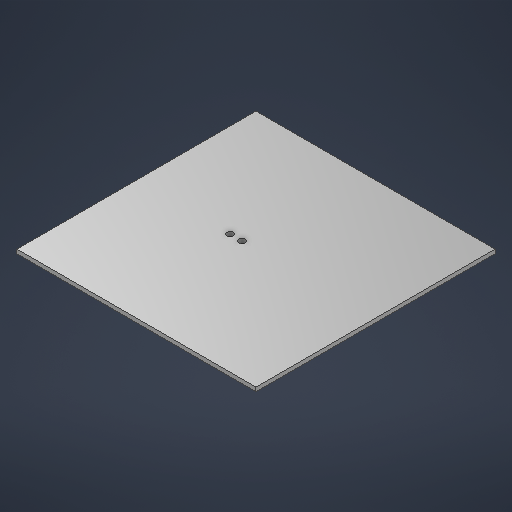
# Autodesk Inventor part: PlataformaLoadCell
Saved by Autodesk Inventor 2027 (Build 310192060, 192F)
## iProperties
Created: 2026-09-27
Part Number: PlataformaLoadCell
Material: PC/ABS Plastic
Document SubType Name: Modeling
Designer: notra
Density: 1.1 g/cm^3
Appearance: Smooth - White
Mass: 229.26 g
Surface Area: 860.831 cm^2
Volume: 208.419 cm^3
Author: notra
Autodesk Inventor part; units mm, degrees
ref_plane "YZ Plane" through (0, 0, 0) normal (1, 0, 0) x (0, 1, 0)
ref_plane "XZ Plane" through (0, 0, 0) normal (0, 1, 0) x (-1, 0, 0)
ref_plane "XY Plane" through (0, 0, 0) normal (0, 0, 1) x (1, 0, 0)
sketch "Sketch1" plane through (0, 0, 0) normal (0, 1, 0) x (-1, 0, 0)
  line L0 (-150, 150) -> (150, 150)
  line L1 (150, 150) -> (150, -150)
  line L2 (150, -150) -> (-150, -150)
  line L3 (-150, -150) -> (-150, 150)
  line L4 (-150, 150) -> (150, -150) construction
  line L5 (150, 150) -> (-150, -150) construction
  line L6 (150, 0) -> (-150, 0) construction
  line L7 (0, 150) -> (0, -150) construction
  line L8 (37.5, 6.35) -> (-37.5, 6.35) construction
  line L9 (-37.5, 6.35) -> (-37.5, -6.35) construction
  line L10 (-37.5, -6.35) -> (37.5, -6.35) construction
  line L11 (37.5, -6.35) -> (37.5, 6.35) construction
  line L12 (37.5, 6.35) -> (-37.5, -6.35) construction
  line L13 (-37.5, 6.35) -> (37.5, -6.35) construction
  circle A0 centre (32.5, 0) radius 2
  circle A1 centre (17.5, 0) radius 2
  circle A2 centre (-32.5, 0) radius 2 construction
  circle A3 centre (-17.5, 0) radius 2 construction
  line L14 (30.5, 0) -> (19.5, 0) construction
  line L15 (42.5, 13.75) -> (7.5, 13.75)
  line L16 (7.5, 13.75) -> (7.5, -13.75)
  line L17 (7.5, -13.75) -> (42.5, -13.75)
  line L18 (42.5, -13.75) -> (42.5, 13.75)
  line L19 (42.5, 13.75) -> (7.5, -13.75) construction
  line L20 (7.5, 13.75) -> (42.5, -13.75) construction
  circle A4 centre (32.5, 0) radius 4
  circle A5 centre (17.5, 0) radius 4
  point P0 (0, 0)
  point P1 (37.5, 0)
  point P2 (25, 0)
  dimension "d4" = 4
  dimension "d7" = 4
  dimension "d0" = 300
  dimension "d1" = 300
  dimension "d2" = 75
  dimension "d3" = 12.7
  dimension "d5" = 5
  dimension "d8" = 15
  dimension "d9" = 35
  dimension "d10" = 27.5
  dimension "d15" = 8
  dimension "d16" = 8
  constraints: 42 end point, 12 midpoint, 6 parallel, 4 centre point, 4 point on line, 3 horizontal, 3 perpendicular, 2 coincident, 2 horizontal alignment, 2 symmetric about line, 6 other
  measures "d0" distance of L1.end L2.end
  measures "d1" distance of L0.end L1.end
  measures "d2" distance of L10.end L9.end
  measures "d3" distance of L9.end L8.end
  measures "d5" distance of point (37.5, 0) point (32.5, 0)
  measures "d8" distance of point (17.5, 0) point (32.5, 0)
  measures "d9" distance of L17.end L16.end
  measures "d10" distance of L16.end L15.end
  measures "d15" diameter of A4
  measures "d16" diameter of A5
extrude "Extrusion1" add sketch "Sketch1" along normal blind 5 contours L0 L1 L2 L3 | L18 L17 L16 L15 | A4 | A5
extrude "Extrusion2" add sketch "Sketch1" against normal blind 10 contours L18 L17 L16 L15 | A4 | A5
extrude "Extrusion3" cut sketch "Sketch1" along normal blind 10 contours A4 | A5
fillet "Fillet1" radius 2 4 edges at (-42.5, 0, 0) (-25, 0, 13.75) (-25, 0, -13.75) (-7.5, 0, 0)
sketch "Sketch2" plane through (-42.5, -10, 13.75) normal (0, 0, 1) x (1, 0, 0)
  line L0 (0, 8) -> (35, 8) projected
  line L1 (0, 8) -> (0, 0) projected
  line L2 (35, 0) -> (0, 0) projected
  line L3 (35, 8) -> (35, 0) projected
  line L4 (10, 8) -> (10, 0) construction
  line L5 (7, 5.6) -> (13, 5.6)
  line L6 (13, 5.6) -> (13, 2.4)
  line L7 (13, 2.4) -> (7, 2.4)
  line L8 (7, 2.4) -> (7, 5.6)
  line L9 (7, 5.6) -> (13, 2.4) construction
  line L10 (13, 5.6) -> (7, 2.4) construction
  line L11 (0, 4) -> (10, 4) construction
  line L12 (35, 0) -> (0, 0) projected
  line L13 (17.5, 0) -> (17.5, 8) construction
  line L14 (28, 5.6) -> (22, 5.6)
  line L15 (22, 5.6) -> (22, 2.4)
  line L16 (22, 2.4) -> (28, 2.4)
  line L17 (28, 2.4) -> (28, 5.6)
  line L18 (28, 5.6) -> (22, 2.4) construction
  line L19 (22, 5.6) -> (28, 2.4) construction
  point P0 (42.5, 10)
  point P1 (25, 4)
  dimension "d20" = 10
  dimension "d21" = 6
  dimension "d22" = 3.2
  constraints: 30 end point, 6 midpoint, 5 symmetric about line, 3 parallel, 2 horizontal, 1 perpendicular
  measures "d20" distance between parallel lines of L1 L4
  measures "d21" distance of L6.end L7.end
  measures "d22" distance of L5.end L6.end
extrude "Extrusion4" cut sketch "Sketch2" against normal blind 16.75 contours L5 L6 L7 L8 | L17 L16 L15 L14
body "Solid1"
